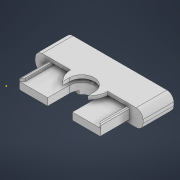
# Autodesk Inventor part: syringe_fitter
Saved by Autodesk Inventor 2022 (Build 260153000, 153)
## iProperties
Created: 2023-04-21
Part Number: syringe_fitter
Material: Generic
Document SubType Name: Modeling
Designer: Jakob Saugbjerg
Density: 1 g/cm^3
Appearance: Default
Author: Jakob Saugbjerg
Autodesk Inventor part; units mm, degrees
ref_plane "YZ Plane" through (0, 0, 0) normal (1, 0, 0) x (0, 1, 0)
ref_plane "XZ Plane" through (0, 0, 0) normal (0, 1, 0) x (-1, 0, 0)
ref_plane "XY Plane" through (0, 0, 0) normal (0, 0, 1) x (1, 0, 0)
sketch "Sketch13" plane through (0, 0, 0) normal (0, 0, 1) x (1, 0, 0)
  line L0 (0, 0) -> (63, 0)
  line L1 (63, 0) -> (63, 10)
  line L2 (63, 10) -> (0, 10)
  line L3 (0, 10) -> (0, 0)
  dimension "d38" = 63
  dimension "d39" = 10
  constraints: 8 end point, 2 parallel, 1 horizontal, 1 perpendicular
  measures "d38" distance of L2.end L1.end
  measures "d39" distance of L1.end L0.end
extrude "Extrusion8" add sketch "Sketch13" along normal blind 35
sketch "Sketch15" plane through (0, 10, 0) normal (0, 1, 0) x (1, 0, 0)
  line L0 (63, -35) -> (0, -35) projected
  line L1 (31.5, -35) -> (31.5, -22.25)
  circle A0 centre (31.5, -22.25) radius 7.25
  line L2 (44, -35) -> (24.25, -35)
  line L3 (24.25, -35) -> (24.25, -22.25)
  line L4 (38.75, -22.25) -> (38.75, -35)
  point P0 (0, 0)
  dimension "d42" = 12.75
  dimension "d43" = 14.5
  constraints: 8 end point, 2 point on circle, 2 point on line, 1 centre point, 1 coincident, 1 midpoint, 1 perpendicular, 1 vertical
  measures "d42" distance of L1.start L1.end
  measures "d43" diameter of A0
extrude "Extrusion9" cut sketch "Sketch15" against normal blind 35
sketch "Sketch16" plane through (0, 10, 0) normal (0, 1, 0) x (1, 0, 0)
  line L0 (0, -35) -> (24.25, -35) projected
  line L1 (0, -35) -> (63, -35)
  line L2 (63, -35) -> (63, -18)
  line L3 (63, -18) -> (0, -18)
  line L4 (0, -18) -> (0, -35)
  point P0 (0, 0)
  dimension "d46" = 63
  dimension "d47" = 17
  constraints: 8 end point, 2 parallel, 1 horizontal, 1 perpendicular
  measures "d46" distance of L3.end L2.end
  measures "d47" distance of L2.end L1.end
extrude "Extrusion10" cut sketch "Sketch16" against normal blind 2
sketch "Sketch17" plane through (0, 0, 0) normal (0, -1, 0) x (1, 0, 0)
  line L0 (0, 35) -> (24.25, 35) projected
  line L1 (0, 35) -> (63, 35)
  line L2 (63, 35) -> (63, 18)
  line L3 (63, 18) -> (0, 18)
  line L4 (0, 18) -> (0, 35)
  dimension "d71" = 63
  dimension "d72" = 17
  constraints: 8 end point, 2 parallel, 1 horizontal, 1 perpendicular
  measures "d71" distance of L2.end L3.end
  measures "d72" distance of L1.end L2.end
extrude "Extrusion11" cut sketch "Sketch17" against normal blind 2
sketch "Sketch19" plane through (0, 0, 35) normal (0, 0, 1) x (1, 0, 0)
  line L0 (24.25, 8) -> (0, 8) projected
  line L1 (9.5, 8) -> (53.5, 8)
  line L2 (53.5, 8) -> (53.5, 6.2)
  line L3 (53.5, 6.2) -> (9.5, 6.2)
  line L4 (9.5, 6.2) -> (9.5, 8)
  point P0 (0, 0)
  dimension "d68" = 1.8
  constraints: 8 end point, 2 parallel, 1 horizontal, 1 perpendicular, 1 point on line
  measures "d68" distance of L1.end L2.end
extrude "Extrusion12" cut sketch "Sketch19" against normal blind 33
fillet "Fillet5" radius 2 2 edges at (9.5, 7.1, 35) (53.5, 7.1, 35)
sketch "Sketch20" plane through (0, 0, 35) normal (0, 0, 1) x (1, 0, 0)
  line L0 (63, 8) -> (38.75, 8) projected
  line L1 (7.5, 2) -> (55.5, 2)
  line L2 (55.5, 2) -> (55.5, 8)
  line L3 (55.5, 8) -> (7.5, 8)
  line L4 (7.5, 8) -> (7.5, 2)
  line L5 (7.5, 2) -> (55.5, 8) construction
  line L6 (55.5, 2) -> (7.5, 8) construction
  line L7 (7.5, 8) -> (0, 8)
  line L8 (0, 8) -> (0, 2)
  line L9 (0, 2) -> (7.5, 2)
  line L10 (7.5, 2) -> (7.5, 8)
  line L11 (38.75, 2) -> (63, 2) projected
  line L12 (55.5, 8) -> (63, 8)
  line L13 (63, 8) -> (63, 2)
  line L14 (63, 2) -> (55.5, 2)
  line L15 (55.5, 2) -> (55.5, 8)
  point P0 (0, 0)
  point P1 (31.5, 5)
  point P2 (55.5, 2)
  dimension "d58" = 48
  constraints: 28 end point, 6 parallel, 3 horizontal, 3 perpendicular, 2 midpoint, 1 point on line
  measures "d58" distance of L3.end L2.end
extrude "Extrusion13" cut sketch "Sketch20" against normal blind 17 contours L13 L11 L2 L0 | L4 L9 L8 L7
fillet "Fillet6" radius 1 4 edges at (55.5, 2, 26.5) (55.5, 8, 26.5) (7.5, 8, 26.5) (7.5, 2, 26.5)
sketch "Sketch21" plane through (0, 0, 0) normal (0, 0, -1) x (-1, 0, 0)
  spline S0 degree 2 poles (-42.2842, 4.6452) (-42.2842, 4.4254) (-42.425, 4.05) (-42.5534, 3.9116) knots 0 0 0 1 2 2 2
  spline S1 degree 2 poles (-42.5534, 3.9116) (-42.6819, 3.7733) (-43.0647, 3.6128) (-43.3019, 3.6128) knots 0 0 0 1 2 2 2
  spline S2 degree 2 poles (-43.3019, 3.6128) (-43.5192, 3.6128) (-43.9441, 3.7091) (-44.0997, 3.7857) knots 0 0 0 1 2 2 2
  line L0 (-44.0997, 3.7857) -> (-44.0997, 4.2179)
  line L1 (-44.0997, 4.2179) -> (-44.07, 4.2179)
  spline S3 degree 2 poles (-44.07, 4.2179) (-44.0231, 4.1833) (-43.8477, 4.0944) (-43.7415, 4.0549) knots 0 0 0 1 2 2 2
  spline S4 degree 2 poles (-43.7415, 4.0549) (-43.6205, 4.0129) (-43.4204, 3.966) (-43.2945, 3.966) knots 0 0 0 1 2 2 2
  spline S5 degree 2 poles (-43.2945, 3.966) (-43.1709, 3.966) (-42.9388, 4.0549) (-42.8548, 4.1512) knots 0 0 0 1 2 2 2
  spline S6 degree 2 poles (-42.8548, 4.1512) (-42.7782, 4.2426) (-42.6992, 4.4847) (-42.6992, 4.6477) knots 0 0 0 1 2 2 2
  spline S7 degree 2 poles (-42.6992, 4.6477) (-42.6992, 4.8107) (-42.7881, 5.0182) (-42.8721, 5.0874) knots 0 0 0 1 2 2 2
  spline S8 degree 2 poles (-42.8721, 5.0874) (-42.9585, 5.1639) (-43.2154, 5.2282) (-43.371, 5.2282) knots 0 0 0 1 2 2 2
  spline S9 degree 2 poles (-43.371, 5.2282) (-43.539, 5.2282) (-43.8724, 5.1763) (-43.9737, 5.1541) knots 0 0 0 1 2 2 2
  line L2 (-43.9737, 5.1541) -> (-43.9737, 6.725)
  line L3 (-43.9737, 6.725) -> (-42.3015, 6.725)
  line L4 (-42.3015, 6.725) -> (-42.3015, 6.3668)
  line L5 (-42.3015, 6.3668) -> (-43.581, 6.3668)
  line L6 (-43.581, 6.3668) -> (-43.581, 5.5542)
  spline S10 degree 2 poles (-43.581, 5.5542) (-43.5069, 5.5641) (-43.3636, 5.5715) (-43.3043, 5.5715) knots 0 0 0 1 2 2 2
  spline S11 degree 2 poles (-43.3043, 5.5715) (-43.0697, 5.5715) (-42.7461, 5.4949) (-42.5979, 5.3813) knots 0 0 0 1 2 2 2
  spline S12 degree 2 poles (-42.5979, 5.3813) (-42.4472, 5.2677) (-42.2842, 4.9219) (-42.2842, 4.6452) knots 0 0 0 1 2 2 2
  line L7 (-37.8851, 3.677) -> (-37.8851, 5.0009)
  spline S13 degree 2 poles (-37.8851, 5.0009) (-37.8851, 5.159) (-37.9098, 5.4282) (-37.9493, 5.5023) knots 0 0 0 1 2 2 2
  spline S14 degree 2 poles (-37.9493, 5.5023) (-37.9889, 5.5838) (-38.1395, 5.6629) (-38.2704, 5.6629) knots 0 0 0 1 2 2 2
  spline S15 degree 2 poles (-38.2704, 5.6629) (-38.389, 5.6629) (-38.6607, 5.5172) (-38.804, 5.3788) knots 0 0 0 1 2 2 2
  spline S16 degree 2 poles (-38.804, 5.3788) (-38.8015, 5.3443) (-38.7966, 5.2479) (-38.7966, 5.1837) knots 0 0 0 1 2 2 2
  line L8 (-38.7966, 5.1837) -> (-38.7966, 3.677)
  line L9 (-38.7966, 3.677) -> (-39.1819, 3.677)
  line L10 (-39.1819, 3.677) -> (-39.1819, 5.0009)
  spline S17 degree 2 poles (-39.1819, 5.0009) (-39.1819, 5.159) (-39.2066, 5.4282) (-39.2461, 5.5023) knots 0 0 0 1 2 2 2
  spline S18 degree 2 poles (-39.2461, 5.5023) (-39.2856, 5.5838) (-39.4363, 5.6629) (-39.5672, 5.6629) knots 0 0 0 1 2 2 2
  spline S19 degree 2 poles (-39.5672, 5.6629) (-39.6907, 5.6629) (-39.9649, 5.5073) (-40.0933, 5.3862) knots 0 0 0 1 2 2 2
  line L11 (-40.0933, 5.3862) -> (-40.0933, 3.677)
  line L12 (-40.0933, 3.677) -> (-40.4786, 3.677)
  line L13 (-40.4786, 3.677) -> (-40.4786, 5.9642)
  line L14 (-40.4786, 5.9642) -> (-40.0933, 5.9642)
  line L15 (-40.0933, 5.9642) -> (-40.0933, 5.7123)
  spline S20 degree 2 poles (-40.0933, 5.7123) (-39.9426, 5.863) (-39.6462, 6.0284) (-39.4684, 6.0284) knots 0 0 0 1 2 2 2
  spline S21 degree 2 poles (-39.4684, 6.0284) (-39.2659, 6.0284) (-38.9522, 5.8432) (-38.8707, 5.6332) knots 0 0 0 1 2 2 2
  spline S22 degree 2 poles (-38.8707, 5.6332) (-38.6953, 5.8284) (-38.3643, 6.0284) (-38.1716, 6.0284) knots 0 0 0 1 2 2 2
  spline S23 degree 2 poles (-38.1716, 6.0284) (-38.0234, 6.0284) (-37.7814, 5.9371) (-37.6925, 5.8333) knots 0 0 0 1 2 2 2
  spline S24 degree 2 poles (-37.6925, 5.8333) (-37.6011, 5.7296) (-37.4998, 5.4184) (-37.4998, 5.1837) knots 0 0 0 1 2 2 2
  line L16 (-37.4998, 5.1837) -> (-37.4998, 3.677)
  line L17 (-37.4998, 3.677) -> (-37.8851, 3.677)
  line L18 (-35.1632, 3.677) -> (-36.9292, 3.677)
  line L19 (-36.9292, 3.677) -> (-36.9292, 6.725)
  line L20 (-36.9292, 6.725) -> (-36.5241, 6.725)
  line L21 (-36.5241, 6.725) -> (-36.5241, 4.0376)
  line L22 (-36.5241, 4.0376) -> (-35.1632, 4.0376)
  line L23 (-35.1632, 4.0376) -> (-35.1632, 3.677)
  spline S25 degree 2 poles (-32.9476, 3.6227) (-33.1773, 3.6227) (-33.5749, 3.7462) (-33.7058, 3.8153) knots 0 0 0 1 2 2 2
  line L24 (-33.7058, 3.8153) -> (-33.7058, 4.2476)
  line L25 (-33.7058, 4.2476) -> (-33.6861, 4.2476)
  spline S26 degree 2 poles (-33.6861, 4.2476) (-33.6367, 4.208) (-33.5033, 4.1142) (-33.3922, 4.0623) knots 0 0 0 1 2 2 2
  spline S27 degree 2 poles (-33.3922, 4.0623) (-33.2958, 4.0154) (-33.0587, 3.9462) (-32.9327, 3.9462) knots 0 0 0 1 2 2 2
  spline S28 degree 2 poles (-32.9327, 3.9462) (-32.8413, 3.9462) (-32.6314, 3.9882) (-32.582, 4.0228) knots 0 0 0 1 2 2 2
  spline S29 degree 2 poles (-32.582, 4.0228) (-32.5104, 4.0697) (-32.4461, 4.1759) (-32.4461, 4.2846) knots 0 0 0 1 2 2 2
  spline S30 degree 2 poles (-32.4461, 4.2846) (-32.4461, 4.4205) (-32.5943, 4.5613) (-32.7845, 4.6082) knots 0 0 0 1 2 2 2
  spline S31 degree 2 poles (-32.7845, 4.6082) (-32.8586, 4.6255) (-33.0958, 4.6749) (-33.197, 4.7021) knots 0 0 0 1 2 2 2
  spline S32 degree 2 poles (-33.197, 4.7021) (-33.4588, 4.7786) (-33.696, 5.0948) (-33.696, 5.3196) knots 0 0 0 1 2 2 2
  spline S33 degree 2 poles (-33.696, 5.3196) (-33.696, 5.6308) (-33.2291, 6.0186) (-32.8438, 6.0186) knots 0 0 0 1 2 2 2
  spline S34 degree 2 poles (-32.8438, 6.0186) (-32.6536, 6.0186) (-32.2683, 5.9247) (-32.1374, 5.8531) knots 0 0 0 1 2 2 2
  line L26 (-32.1374, 5.8531) -> (-32.1374, 5.4406)
  line L27 (-32.1374, 5.4406) -> (-32.1571, 5.4406)
  spline S35 degree 2 poles (-32.1571, 5.4406) (-32.3053, 5.5591) (-32.666, 5.695) (-32.8512, 5.695) knots 0 0 0 1 2 2 2
  spline S36 degree 2 poles (-32.8512, 5.695) (-33.0414, 5.695) (-33.3032, 5.5344) (-33.3032, 5.3739) knots 0 0 0 1 2 2 2
  spline S37 degree 2 poles (-33.3032, 5.3739) (-33.3032, 5.2282) (-33.1476, 5.0874) (-32.9747, 5.0429) knots 0 0 0 1 2 2 2
  spline S38 degree 2 poles (-32.9747, 5.0429) (-32.8907, 5.0207) (-32.6783, 4.9762) (-32.5622, 4.9491) knots 0 0 0 1 2 2 2
  spline S39 degree 2 poles (-32.5622, 4.9491) (-32.3103, 4.8848) (-32.0534, 4.5909) (-32.0534, 4.3365) knots 0 0 0 1 2 2 2
  spline S40 degree 2 poles (-32.0534, 4.3365) (-32.0534, 4.1883) (-32.1695, 3.9265) (-32.2831, 3.8301) knots 0 0 0 1 2 2 2
  spline S41 degree 2 poles (-32.2831, 3.8301) (-32.4041, 3.7289) (-32.7129, 3.6227) (-32.9476, 3.6227) knots 0 0 0 1 2 2 2
  line L28 (-29.8996, 5.9642) -> (-31.1296, 2.8347)
  line L29 (-31.1296, 2.8347) -> (-31.5421, 2.8347)
  line L30 (-31.5421, 2.8347) -> (-31.1321, 3.7881)
  line L31 (-31.1321, 3.7881) -> (-31.962, 5.9642)
  line L32 (-31.962, 5.9642) -> (-31.5471, 5.9642)
  line L33 (-31.5471, 5.9642) -> (-30.9221, 4.2698)
  line L34 (-30.9221, 4.2698) -> (-30.2997, 5.9642)
  line L35 (-30.2997, 5.9642) -> (-29.8996, 5.9642)
  line L36 (-28.3953, 5.5517) -> (-28.4151, 5.5517)
  spline S42 degree 2 poles (-28.4151, 5.5517) (-28.4595, 5.5641) (-28.5559, 5.569) (-28.6226, 5.569) knots 0 0 0 1 2 2 2
  spline S43 degree 2 poles (-28.6226, 5.569) (-28.7782, 5.569) (-29.0844, 5.4332) (-29.2228, 5.2998) knots 0 0 0 1 2 2 2
  line L37 (-29.2228, 5.2998) -> (-29.2228, 3.677)
  line L38 (-29.2228, 3.677) -> (-29.6081, 3.677)
  line L39 (-29.6081, 3.677) -> (-29.6081, 5.9642)
  line L40 (-29.6081, 5.9642) -> (-29.2228, 5.9642)
  line L41 (-29.2228, 5.9642) -> (-29.2228, 5.6234)
  spline S44 degree 2 poles (-29.2228, 5.6234) (-29.0128, 5.8111) (-28.6991, 5.9642) (-28.5509, 5.9642) knots 0 0 0 1 2 2 2
  spline S45 degree 2 poles (-28.5509, 5.9642) (-28.4916, 5.9642) (-28.4324, 5.9593) (-28.3953, 5.9519) knots 0 0 0 1 2 2 2
  line L42 (-28.3953, 5.9519) -> (-28.3953, 5.5517)
  line L43 (-27.7037, 3.677) -> (-28.089, 3.677)
  line L44 (-28.089, 3.677) -> (-28.089, 5.9642)
  line L45 (-28.089, 5.9642) -> (-27.7037, 5.9642)
  line L46 (-27.7037, 5.9642) -> (-27.7037, 3.677)
  line L47 (-27.6765, 6.3446) -> (-28.1137, 6.3446)
  line L48 (-28.1137, 6.3446) -> (-28.1137, 6.7448)
  line L49 (-28.1137, 6.7448) -> (-27.6765, 6.7448)
  line L50 (-27.6765, 6.7448) -> (-27.6765, 6.3446)
  line L51 (-25.3424, 3.677) -> (-25.7277, 3.677)
  line L52 (-25.7277, 3.677) -> (-25.7277, 4.9812)
  spline S46 degree 2 poles (-25.7277, 4.9812) (-25.7277, 5.1392) (-25.7573, 5.4109) (-25.8018, 5.4925) knots 0 0 0 1 2 2 2
  spline S47 degree 2 poles (-25.8018, 5.4925) (-25.8487, 5.5789) (-26.0167, 5.6629) (-26.1599, 5.6629) knots 0 0 0 1 2 2 2
  spline S48 degree 2 poles (-26.1599, 5.6629) (-26.3032, 5.6629) (-26.607, 5.5097) (-26.7528, 5.3862) knots 0 0 0 1 2 2 2
  line L53 (-26.7528, 5.3862) -> (-26.7528, 3.677)
  line L54 (-26.7528, 3.677) -> (-27.1381, 3.677)
  line L55 (-27.1381, 3.677) -> (-27.1381, 5.9642)
  line L56 (-27.1381, 5.9642) -> (-26.7528, 5.9642)
  line L57 (-26.7528, 5.9642) -> (-26.7528, 5.7098)
  spline S49 degree 2 poles (-26.7528, 5.7098) (-26.5799, 5.8654) (-26.2464, 6.0284) (-26.0587, 6.0284) knots 0 0 0 1 2 2 2
  spline S50 degree 2 poles (-26.0587, 6.0284) (-25.7228, 6.0284) (-25.3424, 5.5838) (-25.3424, 5.1615) knots 0 0 0 1 2 2 2
  line L58 (-25.3424, 5.1615) -> (-25.3424, 3.677)
  spline S51 degree 2 poles (-24.7199, 3.3114) (-24.6804, 3.2941) (-24.5297, 3.2398) (-24.4334, 3.2176) knots 0 0 0 1 2 2 2
  spline S52 degree 2 poles (-24.4334, 3.2176) (-24.3272, 3.1904) (-24.1469, 3.1583) (-24.0407, 3.1583) knots 0 0 0 1 2 2 2
  spline S53 degree 2 poles (-24.0407, 3.1583) (-23.8628, 3.1583) (-23.6158, 3.2522) (-23.5467, 3.3361) knots 0 0 0 1 2 2 2
  spline S54 degree 2 poles (-23.5467, 3.3361) (-23.48, 3.4201) (-23.4281, 3.6399) (-23.4281, 3.7807) knots 0 0 0 1 2 2 2
  line L59 (-23.4281, 3.7807) -> (-23.4281, 3.9808)
  spline S55 degree 2 poles (-23.4281, 3.9808) (-23.5837, 3.845) (-23.8826, 3.7165) (-24.1074, 3.7165) knots 0 0 0 1 2 2 2
  spline S56 degree 2 poles (-24.1074, 3.7165) (-24.4976, 3.7165) (-24.9595, 4.297) (-24.9595, 4.8428) knots 0 0 0 1 2 2 2
  spline S57 degree 2 poles (-24.9595, 4.8428) (-24.9595, 5.1269) (-24.799, 5.5666) (-24.6656, 5.7222) knots 0 0 0 1 2 2 2
  spline S58 degree 2 poles (-24.6656, 5.7222) (-24.5371, 5.8679) (-24.1839, 6.0284) (-23.9962, 6.0284) knots 0 0 0 1 2 2 2
  spline S59 degree 2 poles (-23.9962, 6.0284) (-23.8184, 6.0284) (-23.559, 5.9445) (-23.4281, 5.8679) knots 0 0 0 1 2 2 2
  line L60 (-23.4281, 5.8679) -> (-23.4059, 5.9642)
  line L61 (-23.4059, 5.9642) -> (-23.0428, 5.9642)
  line L62 (-23.0428, 5.9642) -> (-23.0428, 3.9388)
  spline S60 degree 2 poles (-23.0428, 3.9388) (-23.0428, 3.3559) (-23.5491, 2.8125) (-24.0703, 2.8125) knots 0 0 0 1 2 2 2
  spline S61 degree 2 poles (-24.0703, 2.8125) (-24.2383, 2.8125) (-24.589, 2.8668) (-24.7397, 2.9113) knots 0 0 0 1 2 2 2
  line L63 (-24.7397, 2.9113) -> (-24.7397, 3.3114)
  line L64 (-24.7397, 3.3114) -> (-24.7199, 3.3114)
  line L65 (-23.4281, 4.297) -> (-23.4281, 5.5542)
  spline S62 degree 2 poles (-23.4281, 5.5542) (-23.5714, 5.6234) (-23.8134, 5.6826) (-23.9345, 5.6826) knots 0 0 0 1 2 2 2
  spline S63 degree 2 poles (-23.9345, 5.6826) (-24.2259, 5.6826) (-24.5618, 5.2529) (-24.5618, 4.8503) knots 0 0 0 1 2 2 2
  spline S64 degree 2 poles (-24.5618, 4.8503) (-24.5618, 4.4699) (-24.3074, 4.0722) (-24.0209, 4.0722) knots 0 0 0 1 2 2 2
  spline S65 degree 2 poles (-24.0209, 4.0722) (-23.8702, 4.0722) (-23.5541, 4.1908) (-23.4281, 4.297) knots 0 0 0 1 2 2 2
  spline S66 degree 2 poles (-21.4916, 3.6251) (-22.04, 3.6251) (-22.6426, 4.2402) (-22.6426, 4.8083) knots 0 0 0 1 2 2 2
  spline S67 degree 2 poles (-22.6426, 4.8083) (-22.6426, 5.3665) (-22.0573, 6.0284) (-21.5855, 6.0284) knots 0 0 0 1 2 2 2
  spline S68 degree 2 poles (-21.5855, 6.0284) (-21.3731, 6.0284) (-21.0445, 5.9049) (-20.9235, 5.774) knots 0 0 0 1 2 2 2
  spline S69 degree 2 poles (-20.9235, 5.774) (-20.8, 5.6431) (-20.6691, 5.2652) (-20.6691, 4.991) knots 0 0 0 1 2 2 2
  line L66 (-20.6691, 4.991) -> (-20.6691, 4.7811)
  line L67 (-20.6691, 4.7811) -> (-22.2524, 4.7811)
  spline S70 degree 2 poles (-22.2524, 4.7811) (-22.2524, 4.3834) (-21.8522, 3.961) (-21.4966, 3.961) knots 0 0 0 1 2 2 2
  spline S71 degree 2 poles (-21.4966, 3.961) (-21.3706, 3.961) (-21.1261, 4.0179) (-21.0273, 4.0623) knots 0 0 0 1 2 2 2
  spline S72 degree 2 poles (-21.0273, 4.0623) (-20.9235, 4.1117) (-20.7803, 4.1982) (-20.7333, 4.2377) knots 0 0 0 1 2 2 2
  line L68 (-20.7333, 4.2377) -> (-20.7111, 4.2377)
  line L69 (-20.7111, 4.2377) -> (-20.7111, 3.8178)
  spline S73 degree 2 poles (-20.7111, 3.8178) (-20.7778, 3.7906) (-20.9803, 3.7116) (-21.0594, 3.6893) knots 0 0 0 1 2 2 2
  spline S74 degree 2 poles (-21.0594, 3.6893) (-21.1705, 3.6572) (-21.3533, 3.6251) (-21.4916, 3.6251) knots 0 0 0 1 2 2 2
  spline S75 degree 2 poles (-21.0445, 5.075) (-21.0495, 5.2306) (-21.1137, 5.4579) (-21.1755, 5.5344) knots 0 0 0 1 2 2 2
  spline S76 degree 2 poles (-21.1755, 5.5344) (-21.2421, 5.6209) (-21.4521, 5.7123) (-21.6077, 5.7123) knots 0 0 0 1 2 2 2
  spline S77 degree 2 poles (-21.6077, 5.7123) (-21.7608, 5.7123) (-21.9757, 5.6209) (-22.0647, 5.532) knots 0 0 0 1 2 2 2
  spline S78 degree 2 poles (-22.0647, 5.532) (-22.1511, 5.4406) (-22.24, 5.2208) (-22.2524, 5.075) knots 0 0 0 1 2 2 2
  line L70 (-22.2524, 5.075) -> (-21.0445, 5.075)
  point P0 (0, 0)
  point P1 (-44.3541, 6.7448)
  dimension "d38" = 63
  dimension "d39" = 10
  constraints: 1 other
emboss "Emboss3" sketch "Sketch21" operation cut depth 1 direction (0, 0, 1)
sketch "Sketch22" plane through (0, 0, 35) normal (0, 0, 1) x (1, 0, 0)
  point P0 (0, 0)
sketch "Sketch23" plane through (55.5, 3, 18) normal (1, 0, 0) x (0, 0, -1)
  line L0 (-15, 5) -> (0, 5) projected
  line L1 (-17, -1) -> (-17, 0) projected
  line L2 (0, 5) -> (-17, 5)
  line L3 (-17, 5) -> (-17, -1)
  line L4 (-17, -1) -> (0, -1)
  line L5 (0, -1) -> (0, 5)
  point P0 (18, -3)
  point P1 (-15, 5)
  constraints: 8 end point, 2 parallel, 1 horizontal, 1 perpendicular
extrude "Extrusion14" cut sketch "Sketch23" against normal blind 0.2
sketch "Sketch26" plane through (9.5, 6.2, 2) normal (0, 1, 0) x (1, 0, 0)
  arc A0 (16.1263, -16) -> (14.75, -20.25) centre (22, -20.25) ccw projected
  circle A1 centre (22, -20.25) radius 8.5
  line L0 (13.5, -20.25) -> (30.5, -20.25)
  line L1 (30.5, -20.25) -> (30.5, -13)
  line L2 (30.5, -13) -> (13.5, -13)
  line L3 (13.5, -13) -> (13.5, -20.25)
  point P0 (-9.5, 2)
  point P1 (30.5, -20.25)
  point P2 (26.4371, -13)
  point P3 (17.5629, -13)
  dimension "d73" = 17
  dimension "d74" = 7.25
  constraints: 8 end point, 2 parallel, 1 coincident, 1 horizontal, 1 perpendicular, 3 other
  measures "d74" distance of L1.end L0.end
extrude "Extrusion16" [suppressed]
sketch "Sketch24" plane through (7.5, 3, 18) normal (-1, 0, 0) x (0, 0, 1)
  line L0 (0, 5) -> (15, 5) projected
  line L1 (4.25, -1) -> (17, -1) projected
  line L2 (0, 5) -> (17, 5)
  line L3 (17, 5) -> (17, -1)
  line L4 (17, -1) -> (0, -1)
  line L5 (0, -1) -> (0, 5)
  point P0 (-18, -3)
  point P1 (15, 5)
  point P2 (3.5, -1)
  constraints: 8 end point, 2 parallel, 1 horizontal, 1 perpendicular
extrude "Extrusion15" cut sketch "Sketch24" against normal blind 0.2
fillet "Fillet7" radius 4 4 edges at (0, 10, 9) (0, 0, 9) (63, 10, 9) (63, 0, 9)
sketch "Sketch25" plane through (0, 0, 35) normal (0, 0, 1) x (1, 0, 0)
  point P0 (0, 0)
sketch "Sketch27" plane through (0, 0, 35) normal (0, 0, 1) x (1, 0, 0)
  line L0 (53.5, 6.2) -> (9.5, 6.2) projected
  line L1 (9.5, 6.2) -> (53.5, 6.2)
  line L2 (53.5, 6.2) -> (53.5, 8)
  line L3 (53.5, 8) -> (9.5, 8)
  line L4 (9.5, 8) -> (9.5, 6.2)
  point P0 (0, 0)
  constraints: 8 end point, 2 parallel, 1 horizontal, 1 perpendicular
extrude "Extrusion17" cut sketch "Sketch27" against normal blind 20
fillet "Fillet8" [suppressed]
sketch "Sketch28" plane through (31.5, 10, 22.25) normal (0, 1, 0) x (1, 0, 0)
  circle A0 centre (0, 4.25) radius 10.85
  arc A1 (7.25, 0) -> (5.8737, 4.25) centre (0, 0) ccw projected
  line L0 (7.25, 0) -> (7.25, -12.75) projected
  circle A2 centre (0, 0) radius 7.25
  line L1 (-7.25, -12.75) -> (-7.25, 0) projected
  line L2 (-7.25, 0) -> (7.25, 0)
  line L3 (7.25, 0) -> (7.25, -7.25)
  line L4 (7.25, -7.25) -> (-7.25, -7.25)
  line L5 (-7.25, -7.25) -> (-7.25, 0)
  point P0 (-31.5, 22.25)
  point P1 (-7.25, -3.8222)
  point P2 (7.25, -3.8222)
  dimension "d80" = 21.7
  constraints: 8 end point, 2 centre point, 2 parallel, 1 coincident, 1 horizontal, 1 perpendicular, 1 point on circle, 1 point on line
  measures "d80" diameter of A0
extrude "Extrusion18" add sketch "Sketch28" against normal blind 2 contours A0 L0 A1 A2 L1
body "Solid2"
